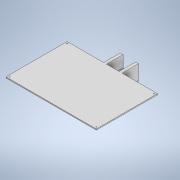
# Autodesk Inventor part: remoteswitchlid
Saved by Autodesk Inventor 2021 (Build 250183000, 183)
## iProperties
Created: 2021-10-23
Part Number: remoteswitchlid
Material: Generic
Document SubType Name: Modeling
Designer: eddys
Density: 1 g/cm^3
Appearance: Default
Author: eddys
Autodesk Inventor part; units mm, degrees
ref_plane "YZ Plane" through (0, 0, 0) normal (1, 0, 0) x (0, 1, 0)
ref_plane "XZ Plane" through (0, 0, 0) normal (0, 1, 0) x (-1, 0, 0)
ref_plane "XY Plane" through (0, 0, 0) normal (0, 0, 1) x (1, 0, 0)
sketch "Sketch1" plane through (0, 0, 0) normal (0, 1, 0) x (-1, 0, 0)
  line L0 (46.5, 31.5) -> (-46.5, 31.5)
  line L1 (-46.5, 31.5) -> (-46.5, -31.5)
  line L2 (-46.5, -31.5) -> (46.5, -31.5)
  line L3 (46.5, -31.5) -> (46.5, 31.5)
  line L4 (46.5, 31.5) -> (-46.5, -31.5) construction
  line L5 (-46.5, 31.5) -> (46.5, -31.5) construction
  point P0 (0, 0)
  dimension "d0" = 63
  dimension "d1" = 93
  constraints: 12 end point, 2 midpoint, 2 parallel, 1 horizontal, 1 perpendicular
  measures "d0" distance of L2.end L0.start
  measures "d1" distance of L1.end L2.end
extrude "Extrusion1" add sketch "Sketch1" along normal blind 1.5
sketch "Sketch2" plane through (0, 1.5, 0) normal (0, 1, 0) x (1, 0, 0)
  circle A0 centre (-44.7, -29.7) radius 0.5
  line L0 (-46.5, 31.5) -> (-46.5, -31.5) projected
  line L1 (-46.5, -31.5) -> (46.5, -31.5) projected
  circle A1 centre (-44.7, 29.7) radius 0.5
  line L2 (46.5, 31.5) -> (-46.5, 31.5) projected
  circle A2 centre (44.7, -29.7) radius 0.5
  line L3 (46.5, -31.5) -> (46.5, 31.5) projected
  circle A3 centre (44.7, 29.7) radius 0.5
  point P0 (0, 0)
  dimension "d4" = 1.8
  dimension "d5" = 1.8
  dimension "d6" = 1
  dimension "d7" = 1.8
  dimension "d8" = 1.8
  dimension "d9" = 1
  dimension "d10" = 1.8
  dimension "d11" = 1.8
  dimension "d12" = 1
  dimension "d13" = 1
  dimension "d14" = 1.8
  dimension "d15" = 1.8
  constraints: 4 centre point
  measures "d4" distance from line of L0 A0.centre
  measures "d5" distance from line of L1 A0.centre
  measures "d6" diameter of A0
  measures "d7" distance from line of L0 A1.centre
  measures "d8" distance from line of L2 A1.centre
  measures "d9" diameter of A1
  measures "d10" distance from line of L1 A2.centre
  measures "d11" distance from line of L3 A2.centre
  measures "d12" diameter of A2
  measures "d13" diameter of A3
  measures "d14" distance from line of L2 A3.centre
  measures "d15" distance from line of L3 A3.centre
extrude "Extrusion2" cut sketch "Sketch2" against normal blind 1.5 contours A0 | A1 | A2 | A3
sketch "Sketch3" plane through (0, 1.5, 0) normal (0, 1, 0) x (1, 0, 0)
  line L0 (46.5, 31.5) -> (-46.5, 31.5) projected
  line L1 (-6, 31.5) -> (7, 31.5)
  line L2 (10, 31.5) -> (10, 28.5)
  line L3 (10, 28.5) -> (-9, 28.5)
  line L4 (-9, 28.5) -> (-9, 31.5)
  line L5 (-46.5, 31.5) -> (-46.5, -31.5) projected
  line L6 (-6, 31.5) -> (-6, 48.5)
  line L7 (-6, 48.5) -> (-9, 48.5)
  line L8 (-9, 48.5) -> (-9, 31.5)
  line L9 (7, 31.5) -> (7, 48.5)
  line L10 (7, 48.5) -> (10, 48.5)
  line L11 (10, 48.5) -> (10, 31.5)
  point P0 (0, 0)
  point P1 (7, 31.5)
  dimension "d18" = 19
  dimension "d20" = 37.5
  dimension "d22" = 3
  dimension "d24" = 3
  dimension "d25" = 20
  dimension "d26" = 20
  dimension "d27" = 3
  dimension "d28" = 17
  dimension "d29" = 3
  constraints: 20 end point, 4 parallel, 1 horizontal, 1 perpendicular, 1 point on line
  measures "d18" distance of L2.end L3.end
  measures "d20" distance between parallel lines of L5 L4
  measures "d22" distance of L6.end L7.end
  measures "d24" distance of L9.end L10.end
  measures "d25" distance between parallel lines of L3 L7
  measures "d26" distance between parallel lines of L3 L10
  measures "d27" distance between parallel lines of L3 L0
  measures "d28" distance between parallel lines of L7 L1
  measures "d29" distance between parallel lines of L8 L6
extrude "Extrusion3" add sketch "Sketch3" against normal blind 12
sketch "Sketch4" plane through (0, -10.5, 0) normal (0, -1, 0) x (1, 0, 0)
  line L0 (-9, -28.5) -> (-9, -48.5) projected
  line L1 (-9, -28.5) -> (10, -28.5)
  line L2 (10, -28.5) -> (10, -48.5)
  line L3 (10, -48.5) -> (-9, -48.5)
  line L4 (-9, -48.5) -> (-9, -28.5)
  point P0 (0, 0)
  constraints: 8 end point, 2 parallel, 1 horizontal, 1 perpendicular
extrude "Extrusion4" add sketch "Sketch4" along normal blind 5
fillet "Fillet1" radius 2 2 edges at (-9, -15.5, -38.5) (10, -15.5, -38.5)
sketch "Sketch5" plane through (-6, 1.5, -48.5) normal (0, 0, -1) x (-1, 0, 0)
  circle A0 centre (-6.5, -15) radius 0.5
  line L0 (3, 0) -> (3, -15) projected
  line L1 (1, -17) -> (-14, -17) projected
  point P0 (-6, -1.5)
  dimension "d35" = 9.5
  dimension "d36" = 2
  dimension "d37" = 1
  constraints: 1 centre point
  measures "d35" distance from line of L0 A0.centre
  measures "d36" distance from line of A0.centre L1
  measures "d37" diameter of A0
extrude "Extrusion5" cut sketch "Sketch5" against normal blind 2
fillet "Fillet2" radius 2 5 edges at (-8.4142, -14.9142, -28.5) (-9, -6.75, -28.5) (9.4142, -14.9142, -28.5) (10, -6.75, -28.5) (0.5, -15.5, -28.5)
fillet "Fillet3" radius 0.5 5 edges at (-27.75, 0, -31.5) (-46.5, 0, 0) (0, 0, 31.5) (28.25, 0, -31.5) (46.5, 0, 0)
body "Solid1"
